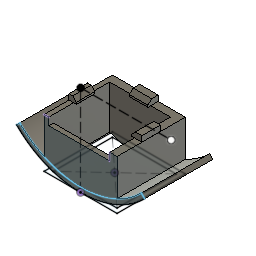
SCD41Chamber (Autodesk Fusion 360 design; units mm, degrees)
Autodesk Fusion 360 part; units mm, degrees
note: some values were not read from the file. Chosen so that the rebuilt part matches the saved one: which face or edge a step refers to. Set by a fixed rule: which sketch regions a step uses.
sketch "Sketch1" plane through (0, 0, 0) normal (0, 1, 0) x (1, 0, 0)
  line L0 (6.85, 6.35) -> (-6.85, 6.35)
  line L1 (-6.85, 6.35) -> (-6.85, -6.35)
  line L2 (-6.85, -6.35) -> (6.85, -6.35)
  line L3 (6.85, -6.35) -> (6.85, 6.35)
  line L4 (6.85, 6.35) -> (-6.85, -6.35) construction
  line L5 (-6.85, 6.35) -> (6.85, -6.35) construction
  line L6 (7.85, -7.35) -> (7.85, 7.35)
  line L7 (7.85, 7.35) -> (-7.85, 7.35)
  line L8 (-7.85, 7.35) -> (-7.85, -7.35)
  line L9 (-7.85, -7.35) -> (7.85, -7.35)
  dimension "d1" = 13.7
  dimension "d2" = 12.7
  dimension "d3" = 1
  constraint horizontal L0
  constraint perpendicular L0 L1
  constraint parallel L0 L2
  constraint parallel L1 L3
  constraint coincident L4 origin
  constraint coincident L5 origin
  measures "d1" distance of L1.end L2.end
  measures "d2" distance of L0.end L1.end
extrude "Extrude1" add sketch "Sketch1" along normal blind 9
sketch "Sketch2" plane through (0, 9, 0) normal (0, 1, 0) x (-1, 0, 0)
  line L0 (-6.85, -6.35) -> (-6.85, 6.35)
  line L1 (-6.85, 6.35) -> (6.85, 6.35)
  line L2 (6.85, 6.35) -> (6.85, -6.35)
  line L3 (6.85, -6.35) -> (-6.85, -6.35)
  line L4 (7.85, 7.35) -> (-7.85, 7.35)
  line L5 (-7.85, 7.35) -> (-7.85, -7.35)
  line L6 (-7.85, -7.35) -> (7.85, -7.35)
  line L7 (7.85, -7.35) -> (7.85, 7.35)
  line L8 (-6.85, 6.35) -> (-6.85, 7.35)
  line L9 (6.85, 6.35) -> (6.85, 7.35)
  constraint coincident L0.end L1.start
  constraint coincident L4 L8.end
  constraint perpendicular L4 L8
  constraint coincident L1.end L2.start
  constraint coincident L4 L9.end
  constraint perpendicular L4 L9
extrude "Extrude2" add sketch "Sketch2" along normal blind 1.6 contours L0 L2 L3 L4 L5 L6 L7 L8 L9
sketch "Sketch3" plane through (0, 10.6, 0) normal (0, 1, 0) x (-1, 0, 0)
  line L0 (6.85, -6.35) -> (-6.85, -6.35)
  line L1 (-6.85, -6.35) -> (-6.85, 7.35)
  line L2 (-6.85, 7.35) -> (-7.85, 7.35)
  line L3 (-7.85, 7.35) -> (-7.85, -7.35)
  line L4 (-7.85, -7.35) -> (7.85, -7.35)
  line L5 (7.85, -7.35) -> (7.85, 7.35)
  line L6 (7.85, 7.35) -> (6.85, 7.35)
  line L7 (6.85, 7.35) -> (6.85, -6.35)
  line L8 (-6.85, 0) -> (-7.35, 0) construction
  line L9 (-7.8685, 2) -> (-6.8315, 2)
  line L10 (-6.8315, 2) -> (-6.8315, -2)
  line L11 (-6.8315, -2) -> (-7.8685, -2)
  line L12 (-7.8685, -2) -> (-7.8685, 2)
  line L13 (-7.8685, 2) -> (-6.8315, -2) construction
  line L14 (-6.8315, 2) -> (-7.8685, -2) construction
  line L15 (6.8315, 2) -> (7.8685, 2)
  line L16 (7.8685, -2) -> (6.8315, -2)
  line L17 (0, -6.35) -> (0, -6.85) construction
  line L18 (-2, -6.3466) -> (2, -6.3466)
  line L19 (2, -6.3466) -> (2, -7.3534)
  line L20 (2, -7.3534) -> (-2, -7.3534)
  line L21 (-2, -7.3534) -> (-2, -6.3466)
  line L22 (-2, -6.3466) -> (2, -7.3534) construction
  line L23 (2, -6.3466) -> (-2, -7.3534) construction
  point P0 (-7.35, 0)
  point P1 (0, -6.85)
  dimension "d8" = 0.5
  dimension "d9" = 4
  dimension "d11" = 180
  dimension "d12" = 0.5
  dimension "d13" = 4
  constraint coincident L1 L8.start
  constraint perpendicular L1 L8
  constraint horizontal L9
  constraint perpendicular L9 L10
  constraint parallel L9 L11
  constraint parallel L10 L12
  constraint coincident L13 P0
  constraint coincident L14 P0
  constraint coincident P0 L8.end
  constraint midpoint L0 L17.start
  constraint perpendicular L0 L17
  constraint horizontal L18
  constraint perpendicular L18 L19
  constraint parallel L18 L20
  constraint parallel L19 L21
  constraint coincident L22 P1
  constraint coincident L23 P1
  constraint coincident P1 L17.end
  measures "d8" distance of L8.start P0
  measures "d9" distance of L9.end L10.end
  measures "d12" distance of L17.start P1
  measures "d13" distance of L19.end L20.end
extrude "Extrude3" add sketch "Sketch3" along normal blind 1.2 contours L0 L18 L19 L21 | L5 L7 L15 L16 | L1 L9 L10 L11
sketch "Sketch4" plane through (0, 0, -6.35) normal (0, 0, 1) x (1, 0, 0)
  line L0 (-6.85, 0) -> (6.85, 0)
  line L1 (6.85, 0) -> (6.85, 10.6)
  line L2 (6.85, 10.6) -> (2, 10.6)
  line L3 (-6.85, 10.6) -> (-6.85, 0)
  line L4 (2, 10.6) -> (-2, 10.6)
  line L5 (2, 10.6) -> (-2, 10.6)
  line L6 (-2, 10.6) -> (-6.85, 10.6)
  constraint coincident L2.end L4.start
extrude "Extrude4" add sketch "Sketch4" along normal blind 0.6
sketch "Sketch5" plane through (-6.85, 0, 0) normal (1, 0, 0) x (0, 0, -1)
  line L0 (-6.35, 0) -> (5.75, 0)
  line L1 (5.75, 10.6) -> (2, 10.6)
  line L2 (2, 10.6) -> (2, 11.8)
  line L3 (2, 11.8) -> (-2, 11.8)
  line L4 (-2, 11.8) -> (-2, 10.6)
  line L5 (-2, 10.6) -> (-7.35, 10.6)
  line L6 (-7.35, 10.6) -> (-7.35, 9)
  line L7 (-7.35, 9) -> (-6.35, 9)
  line L8 (-6.35, 9) -> (-6.35, 0)
  line L9 (-2, 10.6) -> (2, 10.6)
  line L10 (5.75, 0) -> (5.75, 10.6)
  constraint coincident L4.end L5.start
  constraint coincident L1.end L2.start
extrude "Extrude5" add sketch "Sketch5" along normal blind 0.6 contours L2 L3 L4 L9
sketch "Sketch6" plane through (6.85, 0, 0) normal (-1, 0, 0) x (0, 0, 1)
  line L0 (-5.75, 0) -> (6.35, 0)
  line L1 (6.35, 0) -> (6.35, 9)
  line L2 (6.35, 9) -> (7.35, 9)
  line L3 (7.35, 9) -> (7.35, 10.6)
  line L4 (7.35, 10.6) -> (2, 10.6)
  line L5 (-2, 10.6) -> (2, 10.6)
  line L6 (-5.75, 10.6) -> (-5.75, 0)
  line L7 (2, 10.6) -> (-2, 10.6)
  line L8 (-2, 10.6) -> (-5.75, 10.6)
  constraint coincident L4.end L5.end
extrude "Extrude6" add sketch "Sketch6" along normal blind 0.6
chamfer "Chamfer1" distance 0.8 angle 45 1 edges at (-6.25, 11.8, 0)
sketch "Sketch7" plane through (0, 0, 7.35) normal (0, 0, 1) x (1, 0, 0)
  line L0 (-7.85, 0) -> (7.85, 0)
  line L1 (7.85, 0) -> (7.85, 10.6)
  line L2 (7.85, 10.6) -> (6.25, 10.6)
  line L3 (6.25, 9) -> (-6.85, 9)
  line L4 (-6.85, 9) -> (-6.85, 10.6)
  line L5 (-7.85, 10.6) -> (-7.85, 0)
  line L6 (0, 0) -> (0, 19.5) construction
  line L7 (-13.0815, 6.4185) -> (-13.7886, 5.7114)
  line L8 (0, 19.5) -> (19.5, 19.5) construction
  line L9 (13.0815, 6.4185) -> (13.7886, 5.7114)
  line L10 (0, 19.5) -> (19.5, 19.5) construction
  arc A0 (-13.7886, 5.7114) -> (13.7886, 5.7114) centre (0, 19.5) ccw
  arc A1 (-13.0815, 6.4185) -> (13.0815, 6.4185) centre (0, 19.5) ccw
  line L11 (6.25, 10.6) -> (6.25, 9)
  line L12 (-6.85, 10.6) -> (-7.85, 10.6)
  dimension "d23" = 19.5
  dimension "d24" = 39
  dimension "d26" = 135
  dimension "d27" = 45
  constraint coincident L6.start origin
  constraint perpendicular L0 L6
  constraint coincident L6.end L8.start
  constraint horizontal L8
  constraint horizontal L10
  constraint concentric A0 A1
  measures "d23" distance of L6.start L6.end
  measures "d24" diameter of A0
  measures "d26" angle of L7 L8
  measures "d27" angle of L9 L10
extrude "Extrude7" add sketch "Sketch7" against normal up to surface (14.7 mm away) contours L5 L7 A0 A1 | L1 L9 A0 A1
extrude "Extrude8" cut sketch "Sketch7" against normal up to surface (14.7 mm away) contours L0 L5 A0 | L0 L1 A0
extrude "Extrude9" add 1 faces at (0.6667, 11, -6.3466) along direction (0, 0, 1) blind 1.2 and the other way blind 1
extrude "Extrude10" add 1 faces at (6.8315, 11, 0.6667) along direction (-1, 0, 0) blind 1.2 and the other way blind 1
chamfer "Chamfer2" distance 0.8 angle 45 2 edges at (0, 11.8, -5.1466) (5.6315, 11.8, 0)
equation "d24 = ( 19.5 * 2 ) * 1 mm"
